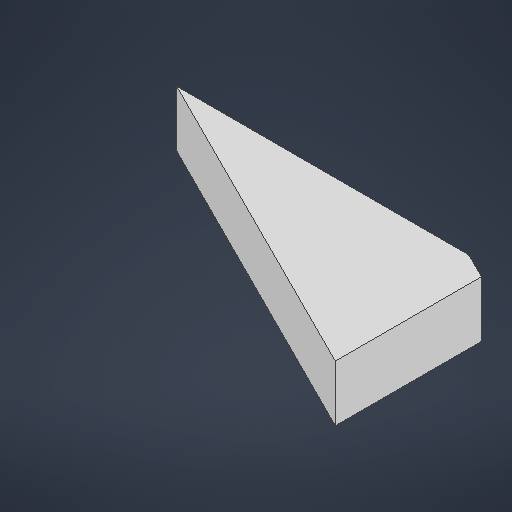
# Autodesk Inventor part: S_2x4x9.503
Saved by Autodesk Inventor 2026 (Build 300175000, 175)
## iProperties
Created: 2025-09-08
Part Number: S_2x4x9.503
Material: Generic
Document SubType Name: Modeling
Designer: trott
Density: 1 g/cm^3
Appearance: Default
Author: trott
Autodesk Inventor part; units mm, degrees
ref_plane "YZ Plane" through (0, 0, 0) normal (1, 0, 0) x (0, 1, 0)
ref_plane "XZ Plane" through (0, 0, 0) normal (0, 1, 0) x (-1, 0, 0)
ref_plane "XY Plane" through (0, 0, 0) normal (0, 0, 1) x (1, 0, 0)
sketch "Sketch1" plane through (0, 0, 0) normal (0, 1, 0) x (-1, 0, 0)
  line L0 (0, 0) -> (-914.4, 0)
  line L1 (-914.4, 0) -> (-914.4, -762)
  line L2 (-914.4, 0) -> (-914.4, 152.4)
  line L3 (0, 0) -> (0, 304.8)
  line L4 (0, 0) -> (-609.6, 0)
  line L5 (-609.6, 0) -> (0, 304.8)
  line L6 (-609.6, 0) -> (-914.4, 152.4)
  line L7 (-914.4, 152.4) -> (-825.5, 152.4)
  line L8 (-825.5, 152.4) -> (-825.5, 0)
  line L9 (-825.5, 0) -> (-825.5, -762)
  line L10 (-825.5, -762) -> (-914.4, -762)
  line L11 (-609.6, 0) -> (-649.3573, -79.5146)
  line L12 (-914.4, 152.4) -> (-954.1573, 72.8854)
  line L13 (-649.3573, -79.5146) -> (-954.1573, 72.8854)
  line L14 (-609.6, 0) -> (-569.8427, -79.5146)
  line L15 (0, 304.8) -> (39.7573, 225.2854)
  line L16 (39.7573, 225.2854) -> (-569.8427, -79.5146)
  point P0 (-410.8136, 0)
  point P1 (0, 205.4068)
  point P2 (-825.5, 8.5568)
  point P3 (-808.3864, 0)
  point P4 (-825.5, 107.95)
  dimension "d0" = 914.4
  dimension "d1" = 762
  dimension "d2" = 152.4
  dimension "d3" = 304.8
  dimension "d4" = 609.6
  dimension "d5" = 88.9
  dimension "d6" = 88.9
  dimension "d7" = 88.9
  dimension "d8" = 88.9
  dimension "d9" = 88.9
  constraints: 34 end point, 6 perpendicular, 3 point on line, 3 vertical, 1 horizontal, 1 parallel
  measures "d0" distance of L0.start L0.end
  measures "d1" distance of L0.end L1.end
  measures "d2" distance of L0.end L2.end
  measures "d3" distance of L0.start L3.end
  measures "d4" distance of L0.start L4.end
  measures "d5" distance of L2.end L7.end
  measures "d6" distance of L4.end L11.end
  measures "d7" distance of L2.end L12.end
  measures "d8" distance of L4.end L14.end
  measures "d9" distance of L3.end L15.end
extrude "Extrusion1" add sketch "Sketch1" along normal blind 38.1 contours L13 L8 L6 L0
body "Solid1"
